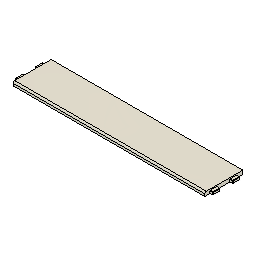
Parametric Centerpiece Template (Autodesk Fusion 360 design; units mm, degrees)
Autodesk Fusion 360 part; units mm, degrees
sketch "Sketch1" plane through (0, 0, 0) normal (0, -1, 0) x (1, 0, 0) in component "DDD Wall Control Center Piece Parametric Template"
  line L0 (125.895, -25) -> (-125.895, -25)
  line L1 (-125.895, -25) -> (-125.895, 25)
  line L2 (-125.895, 25) -> (125.895, 25)
  line L3 (125.895, 25) -> (125.895, -25)
  line L4 (125.895, -25) -> (-125.895, 25) construction
  line L5 (-125.895, -25) -> (125.895, 25) construction
  dimension "d1" = 251.79
  dimension "d2" = 50
  constraint horizontal L0
  constraint perpendicular L0 L1
  constraint parallel L0 L2
  constraint parallel L1 L3
  constraint coincident L4 origin
  constraint coincident L5 origin
  constraint vertical L1
  measures "d1" distance of L1.end L2.end
  measures "d2" distance of L0.end L1.end
extrude "Extrude1" add sketch "Sketch1" against normal blind 5 makes body 1 in component "DDD Wall Control Center Piece Parametric Template"
fillet "Fillet3" radius 2 1 edges at (0, 5, 25) on bodies 1 in component "DDD Wall Control Center Piece Parametric Template"
sketch "Sketch3" plane through (0, 0, 0) normal (1, 0, 0) x (0, 0, 1) in component "DDD Wall Control Center Piece Parametric Template"
  line L0 (-17.25, 0) -> (-7.75, 0)
  line L1 (-7.75, 0) -> (-7.75, -3.5)
  line L2 (-7.75, -3.5) -> (-17.25, -3.5)
  line L3 (-17.25, -3.5) -> (-17.25, 0)
  line L4 (-17.25, 0) -> (-7.75, -3.5) construction
  line L5 (-7.75, 0) -> (-17.25, -3.5) construction
  line L6 (1.75, 0) -> (22.5, 0)
  point P0 (-12.5, -1.75)
  dimension "d165" = 9.5
  dimension "d166" = 3.5
  dimension "d167" = 7.75
  constraint horizontal L0
  constraint perpendicular L0 L1
  constraint parallel L0 L2
  constraint parallel L1 L3
  constraint coincident L4 P0
  constraint coincident L5 P0
  constraint collinear L0 L6
  measures "d165" distance of L1.end L2.end
  measures "d166" distance of L0.start L2.end
  measures "d167" horizontal distance of origin L0.end
extrude "Extrude3" add sketch "Sketch3" along normal blind 4 from surface at 125.895 separate body makes body 2 in component "DDD Wall Control Center Piece Parametric Template"
extrude "Extrude6" add sketch "Sketch3" against normal blind 4 from surface at -125.895 separate body makes body 3 in component "DDD Wall Control Center Piece Parametric Template"
fillet "Fillet4" radius 0.5 16 edges at (129.895, 3.5, -12.5) (129.895, 1.75, -7.75) (127.895, 3.5, -7.75) (127.895, 0, -7.75) (129.895, 0, -12.5) (127.895, 3.5, -17.25) (127.895, 0, -17.25) (129.895, 1.75, -17.25) (-129.895, 3.5, -12.5) (-129.895, 0, -12.5) (-129.895, 1.75, -7.75) (-127.895, 0, -7.75) (-127.895, 3.5, -7.75) (-127.895, 3.5, -17.25) (-127.895, 0, -17.25) (-129.895, 1.75, -17.25) on bodies 2 3 in component "DDD Wall Control Center Piece Parametric Template"
pattern_linear "R-Pattern4" count 2 spacing 26 along (0, 0, 1) of bodies 2 3 makes body 4 at (125.895, 1.1667, 12.0833) makes body 5 at (-125.895, 2.3333, 12.0833) in component "DDD Wall Control Center Piece Parametric Template"
component "DDD Wall Control Center Piece Parametric Template" placed x (1, 0, 0) y (0, 1, 0) z (0, 0, 1) at (0, 0, 0)
equation "d1 = CenterPieceWidthMM"
equation "d2 = CenterPieceDepth"
equation "d3 = -CenterPieceThickness"
equation "CenterPieceWidthUnits = 10" comment "Number of spaces on the wall control pegboard.  Minimum 1,  maximum 14 for vertical wall control panels and 31 for horizonal panels.  Realistically your printer dimensions will determin how big you can make this."
equation "CenterPieceWidthMM = ( CenterPieceWidthUnits * 25.4 mm ) - 2.21 mm" comment "Don't change this.  Change CenterPieceWidthUnits instead.  Final width dimension subtracts 2.21mm from the standard 1\" space between wall control slots to account for the tabs for mouting into the slots"
equation "CenterPieceDepth = 50 mm" comment "Depth measurement from the wall control board extending out into space.  Minimum 17mm to fit at least one mounting tab.  Maximum  ¯\\_(ツ)_/¯"
equation "CenterPieceThickness = 5 mm" comment "Lower measurements make for good shelf-like objects,  taller measurement make for better custom tool holders.  Minimum 5mm to ensure there's enough space for mounting tabs. Maximum  ¯\\_(ツ)_/¯"
equation "CountMountingTabs = 2" comment "Specify the number of mounting tabs to attach a sidepiece"
equation "HowToUse = 0" comment "Save this as a new design seperate from the original to preserve the template.  Then modify as needed for centerpiece divider racks."
equation "d167 = CenterPieceDepth / 2 - 17.25 mm"
equation "d168 = CountMountingTabs"
named bodies: "Center Piece Parametric Template"
